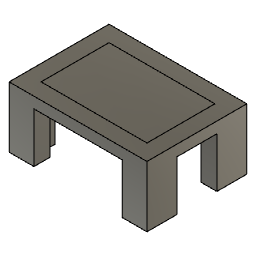
BTS7960 Housing (Autodesk Fusion 360 design; units mm, degrees)
Autodesk Fusion 360 part; units mm, degrees
sketch "Sketch1" plane through (0, 0, 0) normal (0, 0, 1) x (1, 0, 0)
  line L0 (0, 0) -> (69, 0)
  line L1 (69, 0) -> (69, -50)
  line L2 (69, -50) -> (0, -50)
  line L3 (0, -50) -> (0, 0)
  line L4 (8, -8) -> (61, -8)
  line L5 (61, -8) -> (61, -42)
  line L6 (61, -42) -> (8, -42)
  line L7 (8, -42) -> (8, -8)
  dimension "d7" = 69
  dimension "d8" = 50
  dimension "d15" = 34
  dimension "d16" = 53
  dimension "d17" = 8
  dimension "d18" = 8
  constraint horizontal L0
  constraint vertical L1
  constraint horizontal L2
  constraint vertical L3
  constraint coincident L0.start L3.end
  constraint horizontal L4
  constraint vertical L5
  constraint horizontal L6
  constraint vertical L7
  measures "d7" distance of L0.start L0.end
  measures "d8" distance of L0.start L2.end
  measures "d15" distance of L4.start L6.end
  measures "d16" distance of L4.start L4.end
  measures "d17" distance of L0 L4
  measures "d18" distance of L3 L7
extrude "Extrude2" add sketch "Sketch1" along normal blind 30.5 makes body 1
extrude "Extrude1" add sketch "Sketch1" along normal blind 30.5 separate body contours L0 L1 L2 L3 | L4 L5 L6 L7 makes body 2
extrude "Extrude3" cut sketch "Sketch1" along normal blind 25 contours L4 L5 L6 L7 bodies 2
sketch "Sketch3" plane through (0, -50, 0) normal (0, -1, 0) x (1, 0, 0)
  line L0 (0, 0) -> (69, 0)
  line L1 (69, 0) -> (69, 30.5)
  line L2 (69, 30.5) -> (0, 30.5)
  line L3 (0, 30.5) -> (0, 0)
  line L4 (12.4167, 25) -> (56.5833, 25)
  line L5 (56.5833, 25) -> (56.5833, -5.5)
  line L6 (56.5833, -5.5) -> (12.4167, -5.5)
  line L7 (12.4167, -5.5) -> (12.4167, 25)
  dimension "d26" = 44.1667
  dimension "d27" = 30.5
  dimension "d28" = 5.5
  dimension "d32" = 12.4167
  constraint horizontal L4
  constraint vertical L5
  constraint horizontal L6
  constraint vertical L7
  measures "d26" distance of L4.start L4.end
  measures "d27" distance of L4.start L6.end
  measures "d28" distance of L2 L4
  measures "d32" distance of L1 L5
extrude "Extrude4" cut sketch "Sketch3" against normal blind 100 contours L0 L4 L5 L7 | L0 L5 L6 L7 bodies 1 2
sketch "Sketch4" plane through (0, 0, 0) normal (-1, 0, 0) x (0, -1, 0)
  line L0 (0, 0) -> (50, 0)
  line L1 (50, 0) -> (50, 30.5)
  line L2 (50, 30.5) -> (0, 30.5)
  line L3 (0, 30.5) -> (0, 0)
  line L4 (15, 25) -> (35, 25)
  line L5 (35, 25) -> (35, 0)
  line L6 (35, 0) -> (15, 0)
  line L7 (15, 0) -> (15, 25)
  line L8 (50, 0) -> (0, 0)
  line L9 (50, -5.5) -> (50, 25)
  dimension "d36" = 20
  dimension "d37" = 25
  dimension "d40" = 15
  dimension "d43" = 5.5
  constraint horizontal L4
  constraint vertical L5
  constraint horizontal L6
  constraint vertical L7
  measures "d36" distance of L4.start L4.end
  measures "d37" distance of L4.start L6.end
  measures "d40" distance of L5 L9
  measures "d43" distance of L2 L4
extrude "Extrude5" cut sketch "Sketch4" against normal blind 113 contours L0 L4 L5 L6 L7 L8 bodies 1 2
equation "bottom_thickness = 5.5 mm"
equation "side_thickness = 8 mm"
equation "outer_width = inner_width + 2 * side_thickness"
equation "height = 25 mm + bottom_thickness"
equation "outer_length = inner_length + 2 * side_thickness"
equation "inner_length = 53 mm"
equation "d7 = outer_length"
equation "d8 = outer_width"
equation "d9 = height"
equation "inner_width = 34 mm"
equation "d15 = inner_width"
equation "d16 = inner_length"
equation "d17 = side_thickness"
equation "d18 = side_thickness"
equation "d19 = height"
equation "d21 = height - bottom_thickness"
equation "big_side_gap = 5 * inner_length / 6"
equation "big_side_gap_distance = ( outer_length - big_side_gap ) / 2"
equation "extra = 100 mm"
equation "d26 = big_side_gap"
equation "d27 = height"
equation "d28 = bottom_thickness"
equation "d30 = -extra"
equation "d32 = big_side_gap_distance"
equation "small_side_gap_width = 25 mm"
equation "small_side_gap_length = 20 mm"
equation "small_side_gap_depth = side_thickness + 5 mm"
equation "d36 = small_side_gap_length"
equation "d37 = small_side_gap_width"
equation "small_side_gap_distance = ( outer_width - small_side_gap_length ) / 2"
equation "d40 = small_side_gap_distance"
equation "d41 = -small_side_gap_depth - 100 mm"
equation "d43 = bottom_thickness"
equation "cable_dent = 5 mm"
